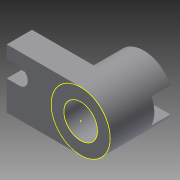
# Autodesk Inventor part: 零件2
Saved by Autodesk Inventor 2014 (Build 180170000, 170)
## iProperties
Created: 2018-11-23
Part Number: 零件2
Material: 常规
Document SubType Name: Modeling
Designer: Administrator
Density: 1 g/cm^3
Appearance: 默认
Author: Administrator
Autodesk Inventor part; units mm, degrees
ref_plane "YZ Plane" through (0, 0, 0) normal (1, 0, 0) x (0, 1, 0)
ref_plane "XZ Plane" through (0, 0, 0) normal (0, 1, 0) x (-1, 0, 0)
ref_plane "XY Plane" through (0, 0, 0) normal (0, 0, 1) x (1, 0, 0)
sketch "草图1" plane through (0, 0, 0) normal (0, 1, 0) x (-1, 0, 0)
  circle A0 centre (0, 0) radius 8
  circle A1 centre (0, 0) radius 14
  dimension "d0" = 16
  dimension "d1" = 28
  constraints: 2 centre point, 2 coincident
  measures "d0" diameter of A0
  measures "d1" diameter of A1
extrude "拉伸1" add sketch "草图1" along normal blind 30
sketch "草图2" plane through (0, 30, 0) normal (0, 1, 0) x (1, 0, 0)
  circle A0 centre (0, 0) radius 14 projected
  line L0 (18.1173, -6) -> (-18.1173, -6)
  line L1 (-18.1173, -6) -> (-18.1173, 6)
  line L2 (-18.1173, 6) -> (18.1173, 6)
  line L3 (18.1173, 6) -> (18.1173, -6)
  line L4 (18.1173, -6) -> (-18.1173, 6) construction
  line L5 (-18.1173, -6) -> (18.1173, 6) construction
  dimension "d4" = 12
  dimension "d5" = 36.2346
  constraints: 12 end point, 2 midpoint, 2 parallel, 1 horizontal, 1 perpendicular
  measures "d4" distance of L0.end L1.end
  measures "d5" distance of L1.end L2.end
extrude "拉伸2" cut sketch "草图2" against normal blind 9 contours A0 L0 L2 | A0 L2 L3 L0 | A0 L0 L1 L2
sketch "草图3" plane through (0, 0, 0) normal (0, -1, 0) x (1, 0, 0)
  circle A0 centre (0, 0) radius 14 projected
  line L0 (0, 14) -> (-35, 14)
  line L1 (0, -14) -> (-35, -14)
  line L2 (-41.9506, 4) -> (-20.5959, 4)
  arc A1 (-29, 0) -> (-29, 8) centre (-29, 4) ccw
  line L3 (-29, 8) -> (-35, 8)
  line L4 (-29, 0) -> (-35, 0)
  line L5 (-35, 14) -> (-35, 8)
  line L6 (-35, 0) -> (-35, -14)
  dimension "d8" = 8
  dimension "d9" = 35
  dimension "d10" = 35
  dimension "d11" = 6
  dimension "d12" = 6
  constraints: 14 end point, 8 perpendicular, 4 point on circle, 4 tangent, 1 centre point, 1 horizontal, 1 parallel, 1 point on line
  measures "d8" diameter of A1
  measures "d9" distance of L0.start L0.end
  measures "d10" distance of L1.start L1.end
  measures "d11" distance of L3.start L3.end
  measures "d12" distance of L0.end L3.end
sketch "草图4" plane through (0, 0, 0) normal (0, -1, 0) x (1, 0, 0)
  circle A0 centre (0, 0) radius 8 projected
  circle A1 centre (0, 0) radius 14 projected
extrude "拉伸3" add sketch "草图3" against normal blind 12 contours A0 L1 L6 L4 A1 L3 L5 L0
sketch "草图5" plane through (0, 12, 0) normal (0, 1, 0) x (1, 0, 0)
  line L0 (-35, 14) -> (-35, 0) projected
  line L1 (-35, 0) -> (-29, 0) projected
  arc A0 (-29, -8) -> (-29, 0) centre (-29, -4) ccw projected
  line L2 (-29, -8) -> (-35, -8) projected
  line L3 (-35, -8) -> (-35, -14) projected
  arc A1 (-29, -10) -> (-29, 2) centre (-29, -4) ccw
  line L4 (-29, 2) -> (-35, 2)
  line L5 (-29, -10) -> (-35, -10)
  dimension "d15" = 12
  constraints: 4 end point, 2 perpendicular, 2 point on circle, 2 point on line, 2 tangent, 1 centre point, 1 coincident
  measures "d15" diameter of A1
extrude "拉伸4" cut sketch "草图5" against normal blind 5
